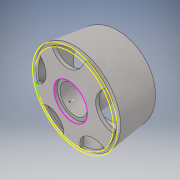
# Autodesk Inventor part: AutomobloxWheel
Saved by Autodesk Inventor 2018 (Build 220112000, 112)
## iProperties
Created: 2019-01-09
Part Number: AutomobloxWheel
Material: Generic
Document SubType Name: Modeling
Designer: 10043883
Density: 1 g/cm^3
Appearance: Weld - Steel Mild
Cost Center: 1B
Author: 10043883
Autodesk Inventor part; units mm, degrees
ref_plane "YZ Plane" through (0, 0, 0) normal (1, 0, 0) x (0, 1, 0)
ref_plane "XZ Plane" through (0, 0, 0) normal (0, 1, 0) x (-1, 0, 0)
ref_plane "XY Plane" through (0, 0, 0) normal (0, 0, 1) x (1, 0, 0)
sketch "Sketch1" plane through (0, 0, 0) normal (0, 0, 1) x (1, 0, 0)
  circle A0 centre (0, 0) radius 5.588
  circle A1 centre (0, 0) radius 6.858
  circle A2 centre (0, 0) radius 15.748
  circle A3 centre (0, 0) radius 17.018
  dimension "d0" = 11.176
  dimension "d1" = 1.27
  dimension "d2" = 8.89
  dimension "d3" = 1.27
  constraints: 4 centre point, 4 coincident
  measures "d0" diameter of A0
  measures "d1" radial gap between concentric circles of A0 A1
  measures "d2" radial gap between concentric circles of A1 A2
  measures "d3" radial gap between concentric circles of A2 A3
extrude "Extrusion1" add sketch "Sketch1" along normal blind 14.478
sketch "Sketch2" plane through (0, 0, 14.478) normal (0, 0, 1) x (1, 0, 0)
  circle A0 centre (0, 0) radius 5.588 projected
  circle A1 centre (0, 0) radius 6.858 projected
  circle A2 centre (0, 0) radius 15.748 projected
  circle A3 centre (0, 0) radius 17.018 projected
extrude "Extrusion2" add sketch "Sketch2" along normal blind 1.27 contours A2
sketch "Sketch4" plane through (0, 0, 14.478) normal (0, 0, 1) x (1, 0, 0)
  point P0 (0, 0)
sketch "Sketch6" plane through (0, 0, 15.748) normal (0, 0, 1) x (1, 0, 0)
  arc A0 (-5.904, 14.5994) -> (5.8746, 14.6117) centre (-0.0172, 16.98) ccw
  arc A1 (5.8746, 14.6117) -> (-5.904, 14.5994) centre (0.0005, -0.0013) ccw
  arc A2 (-12.082, 10.101) -> (-15.7101, -1.105) centre (0.0005, -0.0013) ccw
  arc A3 (-15.7101, -1.105) -> (-12.082, 10.101) centre (-16.1551, 5.2294) ccw
  arc A4 (-13.341, -8.3707) -> (-3.8047, -15.284) centre (0.0005, -0.0013) ccw
  arc A5 (-3.8047, -15.284) -> (-13.341, -8.3707) centre (-9.9665, -13.7498) ccw
  arc A6 (3.8375, -15.2761) -> (13.3594, -8.3428) centre (0.0005, -0.0013) ccw
  arc A7 (13.3594, -8.3428) -> (3.8375, -15.2761) centre (9.9962, -13.729) ccw
  arc A8 (15.7134, -1.0722) -> (12.0619, 10.1261) centre (0.0005, -0.0013) ccw
  arc A9 (12.0619, 10.1261) -> (15.7134, -1.0722) centre (16.1452, 5.2631) ccw
  point P0 (0, 0)
  dimension "d10" = 6.35
  dimension "d13" = 360
  constraints: 20 point on circle, 10 centre point, 2 coincident, 30 other
  measures "d10" radius of A0
sketch "Sketch5" plane through (0, 0, 15.748) normal (0, 0, 1) x (1, 0, 0)
  circle A0 centre (0, 0) radius 17.018 projected
  circle A1 centre (0, 0) radius 15.748 projected
  circle A2 centre (0, 0) radius 6.858 projected
  circle A3 centre (0, 0) radius 15.748 projected
  circle A4 centre (0, 0) radius 6.858 projected
  circle A5 centre (0, 0) radius 15.748 projected
  circle A6 centre (0, 0) radius 15.748 projected
  arc A7 (-14.5821, 5.9465) -> (-14.6389, -5.8053) centre (0, 0) ccw
  arc A8 (-14.5821, 5.9465) -> (-14.6389, -5.8053) centre (0, 0) ccw
  arc A9 (-14.6107, 5.876) -> (-14.6389, -5.8053) centre (0, 0) ccw
  constraints: 7 point on circle, 3 centre point, 2 concentric, 2 other
extrude "Extrusion3" cut sketch "Sketch6" against normal blind 1.27
body "Solid1"
